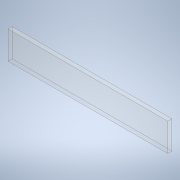
# Autodesk Inventor part: Electronics Side Plate
Saved by Autodesk Inventor 2022 (Build 260153000, 153)
## iProperties
Created: 2022-01-15
Part Number: Electronics Side Plate
Material: Generic
Document SubType Name: Modeling
Designer: merky
Density: 1 g/cm^3
Appearance: Polycarbonate - Clear
Author: merky
Autodesk Inventor part; units mm, degrees
ref_plane "YZ Plane" through (0, 0, 0) normal (1, 0, 0) x (0, 1, 0)
ref_plane "XZ Plane" through (0, 0, 0) normal (0, 1, 0) x (-1, 0, 0)
ref_plane "XY Plane" through (0, 0, 0) normal (0, 0, 1) x (1, 0, 0)
sketch "Sketch1" plane through (0, 0, 0) normal (0, 0, 1) x (1, 0, 0)
  line L0 (0, 0) -> (361.95, 0)
  line L1 (361.95, 0) -> (361.95, 63.5)
  line L2 (361.95, 63.5) -> (0, 63.5)
  line L3 (0, 63.5) -> (0, 0)
  dimension "d0" = 361.95
  dimension "d1" = 63.5
  constraints: 8 end point, 2 parallel, 1 horizontal, 1 perpendicular
  measures "d0" distance of L2.end L1.end
  measures "d1" distance of L1.end L0.end
extrude "Extrusion1" add sketch "Sketch1" along normal blind 9.525
body "Solid1"
